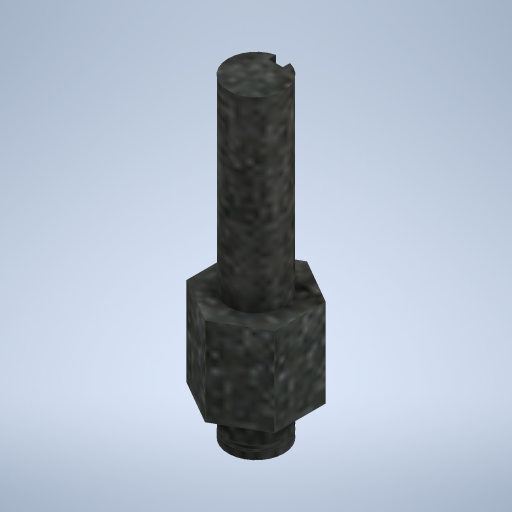
# Autodesk Inventor part: Gear Shaft connector
Saved by Autodesk Inventor 2023 (Build 270158030, 158C)
## iProperties
Created: 2022-10-20
Part Number: Gear Shaft connector
Material: Steel
Document SubType Name: Modeling
Designer: cjj5381
Density: 7.85 g/cm^3
Appearance: Plate
Author: cjj5381
Autodesk Inventor part; units mm, degrees
ref_plane "YZ Plane" through (0, 0, 0) normal (1, 0, 0) x (0, 1, 0)
ref_plane "XZ Plane" through (0, 0, 0) normal (0, 1, 0) x (-1, 0, 0)
ref_plane "XY Plane" through (0, 0, 0) normal (0, 0, 1) x (1, 0, 0)
sketch "Sketch1" plane through (0, 0, 0) normal (0, 1, 0) x (-1, 0, 0)
  line L0 (0, -7.3323) -> (-6.35, -3.6662)
  line L1 (-6.35, -3.6662) -> (-6.35, 3.6662)
  line L2 (-6.35, 3.6662) -> (0, 7.3323)
  line L3 (0, 7.3323) -> (6.35, 3.6662)
  line L4 (6.35, 3.6662) -> (6.35, -3.6662)
  line L5 (6.35, -3.6662) -> (0, -7.3323)
  point P0 (0, 0)
  point P1 (0, 0)
  dimension "d0" = 12.7
  constraints: 12 end point, 1 coincident, 13 other
  measures "d0" distance between parallel lines of L1 L4
extrude "Extrusion1" add sketch "Sketch1" along normal blind 12.7
sketch "Sketch2" plane through (0, 12.7, 0) normal (0, 1, 0) x (1, 0, 0)
  circle A0 centre (0, 0) radius 4
  dimension "d3" = 8
  constraints: 1 centre point, 1 coincident
  measures "d3" diameter of A0
extrude "Extrusion2" add sketch "Sketch2" along normal blind 26.9926 and the other way blind 18.275
sketch "Sketch3" plane through (0, 39.6926, 0) normal (0, 1, 0) x (1, 0, 0)
  line L0 (-1.0287, 4) -> (1.0287, 4)
  line L1 (1.0287, 4) -> (1.0287, 2.8316)
  line L2 (1.0287, 2.8316) -> (-1.0287, 2.8316)
  line L3 (-1.0287, 2.8316) -> (-1.0287, 4)
  line L4 (0, 0) -> (0, 9.4373)
  circle A0 centre (0, 0) radius 4 construction
  circle A1 centre (0, 0) radius 4 construction
  dimension "d6" = 2.0574
  dimension "d8" = 1.1684
  constraints: 10 end point, 2 parallel, 1 horizontal, 1 perpendicular, 1 symmetric about line, 1 tangent, 1 vertical
  measures "d6" distance of L1.end L2.end
  measures "d8" distance of L0.end L1.end
extrude "Extrusion3" cut sketch "Sketch3" against normal up to surface (26.9926 mm away)
sketch "Sketch4" plane through (0, 0, 0) normal (0, 0, 1) x (1, 0, 0)
  line L0 (4, -5.575) -> (4, 0) projected
  line L1 (4, -4.575) -> (3.5, -4.575)
  line L2 (3.5, -4.575) -> (3.5, -3.775)
  line L3 (3.5, -3.775) -> (4, -3.775)
  line L4 (4, -3.775) -> (4, -4.575)
  line L5 (0, -5.575) -> (0, 6.0324)
  line L6 (-4, -5.575) -> (4, -5.575) projected
  point P0 (0, 0)
  point P1 (4, -3.775)
  dimension "d13" = 0.8
  dimension "d14" = 7
  dimension "d16" = 1
  constraints: 10 end point, 2 parallel, 1 horizontal, 1 perpendicular, 1 point on line, 1 vertical
  measures "d13" distance of L1.end L2.end
  measures "d14" diameter of L2 L5
  measures "d16" distance between parallel lines of L6 L1
revolve "Revolution1" cut sketch "Sketch4" angle 360 about axis through (0, -5.575, 0) along (0, 1, 0)
body "Solid1"
